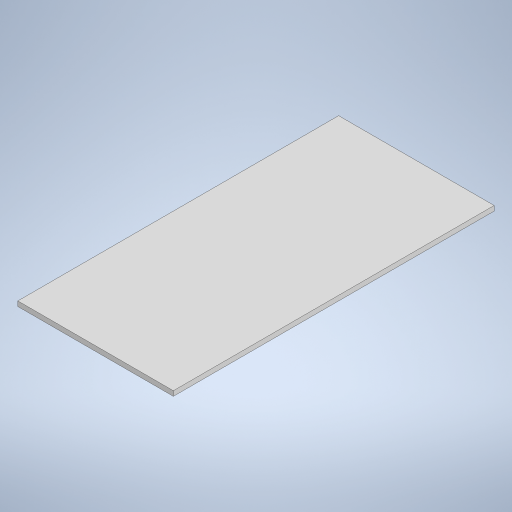
# Autodesk Inventor part: glass bottem container X4
Saved by Autodesk Inventor 2023 (Build 270158000, 158)
## iProperties
Created: 2022-11-22
Part Number: glass bottem container X4
Material: Generic
Document SubType Name: Modeling
Designer: surat
Density: 1 g/cm^3
Appearance: Default
Author: surat
Autodesk Inventor part; units mm, degrees
ref_plane "YZ Plane" through (0, 0, 0) normal (1, 0, 0) x (0, 1, 0)
ref_plane "XZ Plane" through (0, 0, 0) normal (0, 1, 0) x (-1, 0, 0)
ref_plane "XY Plane" through (0, 0, 0) normal (0, 0, 1) x (1, 0, 0)
sketch "Sketch1" plane through (0, 0, 0) normal (0, 1, 0) x (-1, 0, 0)
  line L0 (9.8061, 14.3132) -> (-193.3939, 14.3132)
  line L1 (-193.3939, 14.3132) -> (-193.3939, -404.7868)
  line L2 (-193.3939, -404.7868) -> (9.8061, -404.7868)
  line L3 (9.8061, -404.7868) -> (9.8061, 14.3132)
  point P0 (0, 0)
  dimension "d0" = 203.2
  dimension "d1" = 419.1
  constraints: 8 end point, 2 parallel, 1 horizontal, 1 perpendicular
  measures "d0" distance of L2.end L1.end
  measures "d1" distance of L1.end L0.end
extrude "Extrusion1" add sketch "Sketch1" along normal blind 6.35
body "Solid1"
